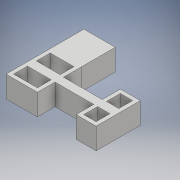
# Autodesk Inventor part: mid_front_Chasis
Saved by Autodesk Inventor 2018.3 (Build 223284000, 284)
## iProperties
Created: 2020-09-12
Part Number: mid_front_Chasis
Material: Generic
Document SubType Name: Modeling
Designer: chris
Density: 1 g/cm^3
Appearance: Default
Author: chris
Autodesk Inventor part; units mm, degrees
ref_plane "YZ Plane" through (0, 0, 0) normal (1, 0, 0) x (0, 1, 0)
ref_plane "XZ Plane" through (0, 0, 0) normal (0, 1, 0) x (-1, 0, 0)
ref_plane "XY Plane" through (0, 0, 0) normal (0, 0, 1) x (1, 0, 0)
sketch "Sketch1" plane through (0, 0, 0) normal (0, 0, 1) x (1, 0, 0)
  line L0 (-60.2002, 26.1718) -> (-60.2002, -26.2038) construction
  line L1 (-60.2002, -26.2038) -> (-23, -26.2038) construction
  line L2 (-23, -26.2038) -> (-23, -5.3034) construction
  line L3 (23, -5.3034) -> (-23, -5.3034) construction
  line L4 (23, -5.3034) -> (23, -26.2034) construction
  line L5 (23, -26.2034) -> (46.6, -26.2034) construction
  line L6 (46.6, -26.2034) -> (46.6, 26.2034) construction
  line L7 (23, 26.2034) -> (46.6, 26.2034) construction
  line L8 (23, 11.4966) -> (23, 26.2034) construction
  line L9 (-8.3, 4.6966) -> (8.3, 4.6966) construction
  line L10 (-23.0002, 26.1718) -> (-23.0002, 11.4966) construction
  line L11 (-23.0002, 26.1718) -> (-60.2002, 26.1718) construction
  line L12 (-27.5, -5.3034) -> (-55.7, -5.3034) construction
  line L13 (-27.5, -5.3034) -> (-27.5, -21.7034) construction
  line L14 (-27.5, -21.7034) -> (-55.7, -21.7034) construction
  line L15 (-55.7, -21.7034) -> (-55.7, -5.3034) construction
  line L16 (42.1, -5.3034) -> (27.5, -5.3034) construction
  line L17 (42.1, -5.3034) -> (42.1, -21.7034) construction
  line L18 (42.1, -21.7034) -> (27.5, -21.7034) construction
  line L19 (27.5, -21.7034) -> (27.5, -5.3034) construction
  line L20 (42.1, 5.3034) -> (42.1, 21.7034) construction
  line L21 (27.5, 5.3034) -> (42.1, 5.3034) construction
  line L22 (27.5, 21.7034) -> (27.5, 5.3034) construction
  line L23 (42.1, 21.7034) -> (27.5, 21.7034) construction
  line L24 (-55.7, 21.7034) -> (-55.7, 5.3034) construction
  line L25 (-27.5, 21.7034) -> (-55.7, 21.7034) construction
  line L26 (-27.5, 5.3034) -> (-27.5, 21.7034) construction
  line L27 (-55.7, 5.3034) -> (-27.5, 5.3034) construction
  line L28 (-60.2002, 26.1718) -> (-23, 26.1718)
  line L29 (-23, -26.2038) -> (-60.2002, -26.2038)
  line L30 (-60.2002, -26.2038) -> (-60.2002, 26.1718)
  line L31 (-55.7, 21.7034) -> (-27.5, 21.7034)
  line L32 (-27.5, 21.7034) -> (-27.5, 5.3034)
  line L33 (-27.5, 5.3034) -> (-55.7, 5.3034)
  line L34 (-55.7, 5.3034) -> (-55.7, 21.7034)
  line L35 (-55.7, -5.3034) -> (-27.5, -5.3034)
  line L36 (-27.5, -5.3034) -> (-27.5, -21.7034)
  line L37 (-27.5, -21.7034) -> (-55.7, -21.7034)
  line L38 (-55.7, -21.7034) -> (-55.7, -5.3034)
  line L39 (-23, 4.6966) -> (23, 4.6966)
  line L40 (23, 26.2034) -> (46.6, 26.2034)
  line L41 (46.6, 26.2034) -> (46.6, -26.2034)
  line L42 (46.6, -26.2034) -> (23, -26.2034)
  line L43 (27.5, 21.7034) -> (42.1, 21.7034)
  line L44 (42.1, 21.7034) -> (42.1, 5.3034)
  line L45 (42.1, 5.3034) -> (27.5, 5.3034)
  line L46 (27.5, 5.3034) -> (27.5, 21.7034)
  line L47 (27.5, -5.3034) -> (42.1, -5.3034)
  line L48 (42.1, -5.3034) -> (42.1, -21.7034)
  line L49 (42.1, -21.7034) -> (27.5, -21.7034)
  line L50 (27.5, -21.7034) -> (27.5, -5.3034)
  line L51 (-23, -5.3034) -> (23, -5.3034)
  line L52 (-23, 26.1718) -> (-23, 4.6966)
  line L53 (-23, -5.3034) -> (-23, -26.2038)
  line L54 (23, -26.2034) -> (23, -5.3034)
  line L55 (23, 4.6966) -> (23, 26.2034)
  point P0 (0, 0)
  point P1 (0, 0)
  point P2 (0, 0)
  constraints: 112 end point, 14 parallel, 7 perpendicular, 6 horizontal, 1 collinear, 1 point on line
extrude "Extrusion1" add sketch "Sketch1" along normal blind 25.4
sketch "Sketch2" plane through (-60.2002, 26.1718, 0) normal (0, 1, 0) x (1, 0, 0)
  line L0 (4.5, -4.5) -> (32.7, -4.5)
  line L1 (32.7, -4.5) -> (32.7, -20.9)
  line L2 (32.7, -20.9) -> (4.5, -20.9)
  line L3 (4.5, -20.9) -> (4.5, -4.5)
  line L4 (37.2, 0) -> (0, 0)
  line L5 (0, 0) -> (0, -25.4)
  line L6 (0, -25.4) -> (37.2, -25.4)
  line L7 (37.2, -25.4) -> (37.2, 0)
  line L8 (0, 0) -> (37.2002, 0) construction
  dimension "d2" = 4.5
  constraints: 16 end point, 4 parallel, 2 perpendicular, 1 horizontal, 3 other
  measures "d2" distance between parallel lines of L0 L4
extrude "Extrusion2" add sketch "Sketch2" along normal blind 40
body "Solid1"
